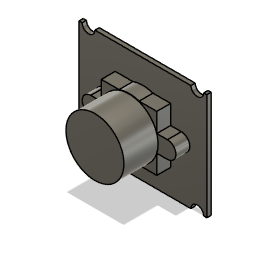
Camera v1 (Autodesk Fusion 360 design; units mm, degrees)
Autodesk Fusion 360 part; units mm, degrees
note: some values were not read from the file. Set by a fixed rule: which sketch regions a step uses.
sketch "Sketch1" plane through (0, 0, 0) normal (0, 1, 0) x (1, 0, 0)
  line L0 (0, 0) -> (-30, 0)
  line L1 (-30, 0) -> (-30, 25)
  line L2 (-30, 25) -> (0, 25)
  line L3 (0, 25) -> (0, 0)
  dimension "d1" = 30
  dimension "d2" = 25
  constraint horizontal L0
  constraint vertical L1
  constraint horizontal L2
  constraint vertical L3
  constraint coincident L0.start L3.end
  measures "d1" distance of L0.start L0.end
  measures "d2" distance of L0.end L1.end
extrude "Extrude1" add sketch "Sketch1" along normal blind 1
move_body "Move1" bodies 1 to x (1, 0, 0) y (0, 0, 1) z (0, -1, 0) at (0, -25, -25)
sketch "Sketch2" plane through (0, 0, -25) normal (0, 0, -1) x (-1, 0, 0)
  line L0 (30, 0) -> (0, 0)
  line L1 (0, 0) -> (0, -25)
  line L2 (0, -25) -> (30, -25)
  line L3 (30, -25) -> (30, 0)
  line L4 (24.1, -25) -> (16.8, -25)
  line L5 (16.8, -25) -> (16.8, -20.5)
  line L6 (16.8, -20.5) -> (24.1, -20.5)
  line L7 (24.1, -20.5) -> (24.1, -25)
  dimension "d6" = 13.2
  dimension "d7" = 7.3
  dimension "d8" = 4.5
  constraint horizontal L4
  constraint vertical L5
  constraint horizontal L6
  constraint vertical L7
  constraint coincident L2 L4.start
  measures "d6" distance of L3 L5
  measures "d7" distance of L5 L7
  measures "d8" distance of L4 L6
extrude "Extrude2" add sketch "Sketch2" along normal blind 3.25 contours L2 L4 L5 L6 L7
sketch "Sketch3" plane through (0, 0, -24) normal (0, 0, 1) x (1, 0, 0)
  line L0 (0, 0) -> (-30, 0)
  line L1 (-30, 0) -> (-30, -25)
  line L2 (-30, -25) -> (0, -25)
  line L3 (0, -25) -> (0, 0)
  line L4 (-21.5, -6) -> (-8.5, -6)
  line L5 (-8.5, -6) -> (-8.5, -19)
  line L6 (-8.5, -19) -> (-21.5, -19)
  line L7 (-21.5, -19) -> (-21.5, -6)
  circle A0 centre (-6, -12.5) radius 2
  circle A1 centre (-24, -12.5) radius 2
  line L8 (-24, -14.5) -> (-21.5, -14.5)
  line L9 (-21.5, -14.5) -> (-21.5, -10.5)
  line L10 (-21.5, -10.5) -> (-24, -10.5)
  line L11 (-24, -10.5) -> (-24, -14.5)
  line L12 (-6, -10.5) -> (-8.5, -10.5)
  line L13 (-8.5, -10.5) -> (-8.5, -14.5)
  line L14 (-8.5, -14.5) -> (-6, -14.5)
  line L15 (-6, -14.5) -> (-6, -10.5)
  circle A2 centre (-15, -12.5) radius 6.91
  dimension "d11" = 19
  dimension "d12" = 19
  dimension "d13" = 21.5
  dimension "d14" = 21.5
  dimension "d15" = 18
  dimension "d18" = 2.5
  dimension "d20" = 13.82
  constraint horizontal L4
  constraint vertical L5
  constraint horizontal L6
  constraint vertical L7
  constraint horizontal L8
  constraint vertical L9
  constraint horizontal L10
  constraint vertical L11
  constraint coincident L7 L9.end
  constraint coincident A1 L8.start
  constraint horizontal L12
  constraint vertical L13
  constraint horizontal L14
  constraint vertical L15
  constraint coincident L5 L13.end
  constraint coincident A0 L12.start
  measures "d11" distance of L2 L4
  measures "d12" distance of L0 L6
  measures "d13" distance of L1 L5
  measures "d14" distance of L3 L7
  measures "d15" distance of A0.centre A1.centre
  measures "d18" distance of L7 A1.centre
  measures "d20" diameter of A2
extrude "Extrude3" add sketch "Sketch3" along normal blind 3.25 contours L4 L7 A2 | L4 A2 | L4 L5 L6 L7 L9 L13 A2 | L4 L5 A2 | L7 L8 L9 L10 A2 | A1 L8 L10 A2 | A1 L11 | A1 L11 | L5 L12 L13 L14 A2 | A0 L12 L14 A2 | L6 L7 A2 | A0 L15 | A0 L15 | L6 A2 | L5 L6 A2
sketch "Sketch4" plane through (0, 0, -20.75) normal (0, 0, 1) x (1, 0, 0)
  line L0 (-8.5, -14.5) -> (-6, -14.5)
  arc A0 (-6, -14.5) -> (-6, -10.5) centre (-6, -12.5) ccw
  line L1 (-6, -10.5) -> (-8.5, -10.5)
  line L2 (-8.5, -10.5) -> (-8.5, -6)
  line L3 (-8.5, -6) -> (-12.6552, -6)
  arc A1 (-12.6552, -6) -> (-17.3448, -6) centre (-15, -12.5) ccw
  line L4 (-17.3448, -6) -> (-21.5, -6)
  line L5 (-21.5, -6) -> (-21.5, -10.5)
  line L6 (-21.5, -10.5) -> (-24, -10.5)
  arc A2 (-24, -10.5) -> (-24, -14.5) centre (-24, -12.5) ccw
  line L7 (-24, -14.5) -> (-21.5, -14.5)
  line L8 (-21.5, -14.5) -> (-21.5, -19)
  line L9 (-21.5, -19) -> (-17.3448, -19)
  arc A3 (-17.3448, -19) -> (-12.6552, -19) centre (-15, -12.5) ccw
  line L10 (-12.6552, -19) -> (-8.5, -19)
  line L11 (-8.5, -19) -> (-8.5, -14.5)
  circle A4 centre (-15, -12.5) radius 6.8007
  constraint concentric A1 A4
  constraint coincident L5.end A4
extrude "Extrude4" add sketch "Sketch4" along normal blind 8 contours A4
sketch "Sketch5" plane through (0, 0, -25) normal (0, 0, -1) x (-1, 0, 0)
  line L0 (16.8, -25) -> (16.8, -20.5)
  line L1 (16.8, -20.5) -> (24.1, -20.5)
  line L2 (24.1, -20.5) -> (24.1, -25)
  line L3 (24.1, -25) -> (30, -25)
  line L4 (30, -25) -> (30, 0)
  line L5 (30, 0) -> (0, 0)
  line L6 (0, 0) -> (0, -25)
  line L7 (0, -25) -> (16.8, -25)
  circle A0 centre (2.25, 0) radius 1.5
  circle A1 centre (27.75, 0) radius 1.5
  circle A2 centre (2.25, -25) radius 1.5
  circle A3 centre (27.75, -25) radius 1.5
  dimension "d25" = 3
  dimension "d26" = 2.25
  dimension "d27" = 3
  dimension "d28" = 2.25
  dimension "d29" = 3
  dimension "d30" = 3
  dimension "d31" = 2.25
  dimension "d32" = 2.25
  constraint coincident L5 A0.centre
  constraint coincident L5 A1.centre
  constraint coincident L7 A2.centre
  constraint coincident L3 A3.centre
  measures "d25" diameter of A0
  measures "d26" distance of L6 A0.centre
  measures "d27" diameter of A1
  measures "d28" distance of L4 A1.centre
  measures "d29" diameter of A2
  measures "d30" diameter of A3
  measures "d31" distance of L6 A2.centre
  measures "d32" distance of L4 A3.centre
extrude "Extrude5" cut sketch "Sketch5" against normal blind 3 contours L7 A2 | L3 A3 | L5 A0 | L5 A1 picked at (2.2874, -24.5014) picked at (27.6014, -24.0139) picked at (2.75, -0.5633) picked at (28.1812, -0.7691)
